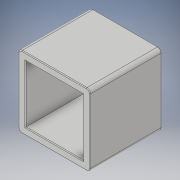
# Autodesk Inventor part: 遙控器盒
Saved by Autodesk Inventor 2019 (Build 230136000, 136)
## iProperties
Created: 2019-02-17
Part Number: 遙控器盒
Material: 一般
Document SubType Name: Modeling
Designer: j13tw
Density: 1 g/cm^3
Appearance: 預設
Author: j13tw
Autodesk Inventor part; units mm, degrees
ref_plane "YZ Plane" through (0, 0, 0) normal (1, 0, 0) x (0, 1, 0)
ref_plane "XZ Plane" through (0, 0, 0) normal (0, 1, 0) x (-1, 0, 0)
ref_plane "XY Plane" through (0, 0, 0) normal (0, 0, 1) x (1, 0, 0)
sketch "草圖1" plane through (0, 0, 0) normal (0, 0, 1) x (1, 0, 0)
  line L0 (-50, 50) -> (50, 50)
  line L1 (50, 50) -> (50, -50)
  line L2 (50, -50) -> (-50, -50)
  line L3 (-50, -50) -> (-50, 50)
  point P0 (0, 0)
  dimension "d0" = 100
  dimension "d1" = 100
  dimension "d2" = 50
  dimension "d3" = 50
  constraints: 8 end point, 2 parallel, 1 horizontal, 1 perpendicular
  measures "d0" distance of L0.start L0.end
  measures "d1" distance of L2.end L0.start
  measures "d2" distance from line of L3 point (0, 0)
  measures "d3" distance from line of L0 point (0, 0)
extrude "擠出1" add sketch "草圖1" along normal blind 100
sketch "草圖2" plane through (0, 0, 100) normal (0, 0, 1) x (1, 0, 0)
  line L0 (-40, 40) -> (40, 40)
  line L1 (40, 40) -> (40, -40)
  line L2 (40, -40) -> (-40, -40)
  line L3 (-40, -40) -> (-40, 40)
  point P0 (0, 0)
  dimension "d6" = 80
  dimension "d7" = 80
  dimension "d8" = 40
  dimension "d9" = 40
  constraints: 8 end point, 2 parallel, 1 horizontal, 1 perpendicular
  measures "d6" distance of L0.start L0.end
  measures "d7" distance of L2.end L0.start
  measures "d8" distance from line of point (0, 0) L3
  measures "d9" distance from line of L2 point (0, 0)
extrude "擠出2" cut sketch "草圖2" against normal blind 90
fillet "圓角1" radius 5 4 edges at (-50, -50, 50) (50, -50, 50) (50, 50, 50) (-50, 50, 50)
fillet "圓角2" radius 1 20 edges at (-48.5355, 48.5355, 100) (-50, 0, 100) (-48.5355, -48.5355, 100) (0, -50, 100) (48.5355, -48.5355, 100) (50, 0, 100) (48.5355, 48.5355, 100) (0, 50, 100) (0, 40, 100) (40, 0, 100) (0, -40, 100) (-40, 0, 100) (-48.5355, 48.5355, 0) (0, 50, 0) (48.5355, 48.5355, 0) (50, 0, 0) (48.5355, -48.5355, 0) (0, -50, 0) (-48.5355, -48.5355, 0) (-50, 0, 0)
